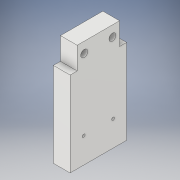
# Autodesk Inventor part: magMount
Saved by Autodesk Inventor 2017 (Build 210142000, 142)
## iProperties
Created: 2017-03-21
Part Number: magMount
Material: Polyethylene, High Density
Document SubType Name: Modeling
Designer: Naga
Density: 0.952 g/cm^3
Appearance: Snow
Author: Naga
Autodesk Inventor part; units mm, degrees
ref_plane "YZ Plane" through (0, 0, 0) normal (1, 0, 0) x (0, 1, 0)
ref_plane "XZ Plane" through (0, 0, 0) normal (0, 1, 0) x (-1, 0, 0)
ref_plane "XY Plane" through (0, 0, 0) normal (0, 0, 1) x (1, 0, 0)
sketch "Sketch1" plane through (0, 0, 0) normal (1, 0, 0) x (0, 1, 0)
  line L0 (0, 0) -> (10, 0)
  line L1 (10, 0) -> (10, -25.4)
  line L2 (10, -25.4) -> (0, -25.4)
  line L3 (0, -25.4) -> (0, 0)
  line L4 (10, 0) -> (0, 0)
  line L5 (0, 0) -> (0, -6.35)
  line L6 (0, -6.35) -> (10, -6.35) construction
  line L7 (10, -6.35) -> (10, 0)
  line L8 (10, -25.4) -> (0, -25.4)
  line L9 (0, -25.4) -> (0, -19.05)
  line L10 (10, -19.05) -> (10, -25.4)
  line L11 (0, -12.7) -> (-19.05, -12.7)
  line L12 (-9.652, -21.59) -> (-28.448, -21.59)
  line L13 (-28.448, -21.59) -> (-28.448, -3.81)
  line L14 (-28.448, -3.81) -> (-9.652, -3.81)
  line L15 (-9.652, -3.81) -> (-9.652, -21.59)
  line L16 (-9.652, -21.59) -> (-28.448, -3.81) construction
  line L17 (-28.448, -21.59) -> (-9.652, -3.81) construction
  line L18 (-28.448, -3.81) -> (-26.67, -3.81)
  line L19 (-26.67, -3.81) -> (-26.67, -6.096)
  circle A0 centre (-26.67, -6.096) radius 0.635
  circle A1 centre (-26.67, -19.304) radius 0.635
  line L20 (-38.1, 0) -> (0, 0)
  line L21 (0, 0) -> (0, -25.4)
  line L22 (0, -25.4) -> (-38.1, -25.4)
  line L23 (-38.1, -25.4) -> (-38.1, 0)
  line L24 (-38.1, 0) -> (0, -25.4) construction
  line L25 (0, 0) -> (-38.1, -25.4) construction
  line L26 (0, 0) -> (10, 0)
  line L27 (10, 0) -> (10, -25.4)
  line L28 (10, -25.4) -> (0, -25.4)
  line L29 (0, -25.4) -> (0, 0)
  line L30 (10, -6.35) -> (5.2248, -6.35)
  circle A2 centre (5.2248, -6.35) radius 1.5875
  line L31 (10, -12.7) -> (5, -12.7)
  circle A3 centre (5.2248, -19.05) radius 1.5875
  dimension "d1" = 25.4
  dimension "d2" = 6.35
  dimension "d3" = 6.35
  dimension "d6" = 19.05
  dimension "d7" = 18.796
  dimension "d8" = 17.78
  dimension "d9" = 1.778
  dimension "d10" = 2.286
  dimension "d11" = 1.27
  dimension "d18" = 4.7752
  dimension "d19" = 3.175
  constraints: 64 end point, 11 parallel, 8 horizontal, 7 perpendicular, 6 midpoint, 4 centre point, 4 point on line, 2 coincident, 2 symmetric about line, 2 other
  measures "d1" distance of L0.end L1.end
  measures "d2" distance of L5.end L4.end
  measures "d3" distance of L8.end L9.end
  measures "d6" distance of L11.start L11.end
  measures "d7" distance of L13.end L14.end
  measures "d8" distance of L12.end L13.end
  measures "d9" distance of L13.end L18.end
  measures "d10" distance of L18.end L19.end
  measures "d11" diameter of A0
  measures "d18" distance of L6.end L30.end
  measures "d19" diameter of A2
extrude "Extrusion1" add sketch "Sketch1" along normal blind 7.5 contours L0 L1 L2 L3 | L3 L22 L23 L20 | L12 L13 L14 L15
sketch "Sketch2" plane through (7.5, 0, 0) normal (1, 0, 0) x (0, 0, -1)
  circle A0 centre (19.304, -26.67) radius 0.635 projected
  circle A1 centre (6.096, -26.67) radius 0.635 projected
  line L0 (0, -38.1) -> (25.4, -38.1) projected
  line L1 (25.4, 10) -> (0, 10) projected
  line L2 (3.175, 0) -> (22.225, 0)
  line L3 (22.225, 0) -> (22.225, 10)
  line L4 (22.225, 10) -> (3.175, 10)
  line L5 (3.175, 10) -> (3.175, 0)
  line L6 (3.175, 0) -> (22.225, 10) construction
  line L7 (22.225, 0) -> (3.175, 10) construction
  line L8 (25.4, -38.1) -> (25.4, 10) projected
  line L9 (0, 0) -> (25.4, 0)
  line L10 (25.4, 0) -> (25.4, 10)
  line L11 (25.4, 10) -> (0, 10)
  line L12 (0, 10) -> (0, 0)
  line L13 (0, 0) -> (25.4, 10) construction
  line L14 (25.4, 0) -> (0, 10) construction
  line L15 (25.4, 10) -> (0, 10) projected
  line L16 (0, 10) -> (0, -38.1) projected
  line L17 (25.4, -38.1) -> (25.4, 10) projected
  point P0 (12.7, 5)
  dimension "d14" = 19.05
  constraints: 24 end point, 4 midpoint, 4 parallel, 2 horizontal, 2 perpendicular, 1 point on line
  measures "d14" distance of L4.end L3.end
extrude "Extrusion2" cut sketch "Sketch2" against normal blind 7.5 contours L12 L1 L5 L9 | L9 L3 L1 L8
body "Solid1"
